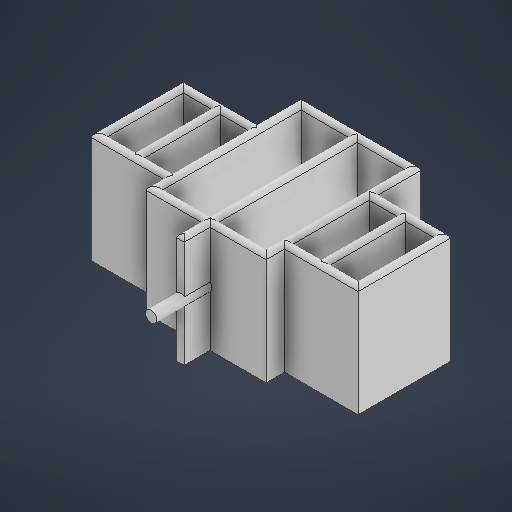
# Autodesk Inventor part: klapy
Saved by Autodesk Inventor 2026.2 (Build 302298010, 298A)
## iProperties
Created: 2026-04-21
Part Number: klapy
Material: Ogólny
Document SubType Name: Modeling
Designer: macie
Density: 1 g/cm^3
Appearance: Domyślna
Author: macie
Autodesk Inventor part; units mm, degrees
ref_plane "YZ Plane" through (0, 0, 0) normal (1, 0, 0) x (0, 1, 0)
ref_plane "XZ Plane" through (0, 0, 0) normal (0, 1, 0) x (-1, 0, 0)
ref_plane "XY Plane" through (0, 0, 0) normal (0, 0, 1) x (1, 0, 0)
sketch "Szkic1" plane through (0, 0, 0) normal (0, 1, 0) x (-1, 0, 0)
  line L0 (16.25, 0) -> (-16.25, 0)
  line L1 (-16.25, 0) -> (-16.25, 2)
  line L2 (-16.25, 2) -> (16.25, 2)
  line L3 (16.25, 2) -> (16.25, 0)
  line L4 (-1, 2) -> (1, 2)
  line L5 (1, 2) -> (1, 49)
  line L6 (1, 49) -> (-1, 49)
  line L7 (-1, 49) -> (-1, 2)
  line L8 (16.25, 2) -> (14.25, 2)
  line L9 (14.25, 2) -> (14.25, 42)
  line L10 (14.25, 42) -> (16.25, 42)
  line L11 (16.25, 42) -> (16.25, 2)
  line L12 (-16.25, 2) -> (-14.25, 2)
  line L13 (-14.25, 2) -> (-14.25, 42)
  line L14 (-14.25, 42) -> (-16.25, 42)
  line L15 (-16.25, 42) -> (-16.25, 2)
  line L16 (14.25, 42) -> (1, 42)
  line L17 (1, 42) -> (1, 40)
  line L18 (1, 40) -> (14.25, 40)
  line L19 (14.25, 40) -> (14.25, 42)
  line L20 (-14.25, 42) -> (-1, 42)
  line L21 (-1, 42) -> (-1, 40)
  line L22 (-1, 40) -> (-14.25, 40)
  line L23 (-14.25, 40) -> (-14.25, 42)
  line L24 (16.25, 37) -> (36.25, 37)
  line L25 (36.25, 37) -> (36.25, 12)
  line L26 (36.25, 12) -> (16.25, 12)
  line L27 (16.25, 12) -> (16.25, 37)
  line L28 (-16.25, 37) -> (-36.25, 37)
  line L29 (-36.25, 37) -> (-36.25, 12)
  line L30 (-36.25, 12) -> (-16.25, 12)
  line L31 (-16.25, 12) -> (-16.25, 37)
  circle A0 centre (0, -31.074) radius 80.074
  line L32 (36.25, 37) -> (34.25, 37)
  line L33 (34.25, 37) -> (34.25, 12)
  line L34 (34.25, 12) -> (36.25, 12)
  line L35 (36.25, 12) -> (36.25, 37)
  line L36 (34.25, 37) -> (16.25, 37)
  line L37 (16.25, 37) -> (16.25, 35)
  line L38 (16.25, 35) -> (34.25, 35)
  line L39 (34.25, 35) -> (34.25, 37)
  line L40 (34.25, 12) -> (16.25, 12)
  line L41 (16.25, 12) -> (16.25, 14)
  line L42 (16.25, 14) -> (34.25, 14)
  line L43 (34.25, 14) -> (34.25, 12)
  line L44 (-16.25, 37) -> (-36.25, 37)
  line L45 (-36.25, 37) -> (-36.25, 35)
  line L46 (-36.25, 35) -> (-16.25, 35)
  line L47 (-16.25, 35) -> (-16.25, 37)
  line L48 (-16.25, 12) -> (-36.25, 12)
  line L49 (-36.25, 12) -> (-36.25, 14)
  line L50 (-36.25, 14) -> (-16.25, 14)
  line L51 (-16.25, 14) -> (-16.25, 12)
  line L52 (-36.25, 35) -> (-34.25, 35)
  line L53 (-34.25, 35) -> (-34.25, 14)
  line L54 (-34.25, 14) -> (-36.25, 14)
  line L55 (-36.25, 14) -> (-36.25, 35)
  line L56 (26.25, 35) -> (24.25, 35)
  line L57 (24.25, 35) -> (24.25, 14)
  line L58 (24.25, 14) -> (26.25, 14)
  line L59 (26.25, 14) -> (26.25, 35)
  line L60 (-24.25, 35) -> (-26.25, 35)
  line L61 (-26.25, 35) -> (-26.25, 14)
  line L62 (-26.25, 14) -> (-24.25, 14)
  line L63 (-24.25, 14) -> (-24.25, 35)
  point P0 (0, 0)
  point P1 (0, 0)
  point P2 (0, 2)
  point P3 (7.625, 40)
  point P4 (7.625, 42)
  point P5 (0, 49)
  point P6 (26.25, 37)
  point P7 (26.25, 14)
  point P8 (1, 42)
  point P9 (1, 48.9938)
  point P10 (-1, 48.9938)
  point P11 (-1, 42)
  point P12 (-16.25, 12)
  point P13 (16.25, 12)
  point P14 (-16.25, 14)
  point P15 (16.25, 14)
  dimension "d0" = 32.5
  dimension "d1" = 2
  dimension "d2" = 2
  dimension "d3" = 49
  dimension "d4" = 40
  dimension "d5" = 2
  dimension "d6" = 2
  dimension "d7" = 2
  dimension "d8" = 20
  dimension "d9" = 20
  dimension "d10" = 25
  dimension "d11" = 25
  dimension "d12" = 160.148
  dimension "d13" = 80.074
  dimension "d14" = 5
  dimension "d15" = 5
  dimension "d16" = 2
  dimension "d17" = 2
  dimension "d18" = 2
  dimension "d19" = 2
  dimension "d20" = 2
  dimension "d21" = 2
  dimension "d22" = 2
  dimension "d23" = 8
  dimension "d24" = 8
  constraints: 128 end point, 32 parallel, 17 point on line, 16 horizontal, 16 perpendicular, 8 midpoint, 1 centre point, 1 coincident
  measures "d0" distance between parallel lines of L1 L3
  measures "d1" distance between parallel lines of L0 L2
  measures "d2" distance between parallel lines of L7 L5
  measures "d3" distance between parallel lines of L6 L0
  measures "d4" distance between parallel lines of L8 L10
  measures "d5" distance between parallel lines of L15 L13
  measures "d6" distance between parallel lines of L11 L9
  measures "d7" distance of point (7.625, 40) point (7.625, 42)
  measures "d8" distance between parallel lines of L11 L25
  measures "d9" distance between parallel lines of L29 L31
  measures "d10" distance between parallel lines of L24 L26
  measures "d11" distance between parallel lines of L30 L28
  measures "d12" diameter of A0
  measures "d13" distance of point (0, 49) A0.centre
  measures "d14" distance between parallel lines of L16 L24
  measures "d15" distance between parallel lines of L20 L28
  measures "d16" distance between parallel lines of L33 L25
  measures "d17" distance between parallel lines of L26 L42
  measures "d18" distance from line of point (26.25, 37) L38
  measures "d19" distance between parallel lines of L46 L28
  measures "d20" distance between parallel lines of L29 L53
  measures "d21" distance between parallel lines of L57 L59
  measures "d22" distance between parallel lines of L61 L63
  measures "d23" distance between parallel lines of L27 L57
  measures "d24" distance between parallel lines of L15 L63
extrude "Wyciągnięcie proste1" add sketch "Szkic1" along normal blind 30 contours L0 L1 L2 L3 | L2 L9 L10 L11 | L15 L14 L13 L2 | L11 L42 L33 L26 | L30 L29 L50 L15 | L2 L7 A0 L5 | L18 L5 L16 L9 | L33 L24 L25 L26 | L13 L20 L7 L22 | L11 L24 L33 L38 | L57 L38 L59 L42 | L46 L29 L28 L15 | L50 L61 L46 L63 | L29 L46 L53 L50
sketch "Szkic2" plane through (1, 0, 42) normal (0, 0, 1) x (1, 0, 0)
  circle A0 centre (-1, 15) radius 1.5
  line L0 (0, 30) -> (15.25, 30) projected
  line L1 (0, 0) -> (0, 30) projected
  point P0 (-1, 0)
  dimension "d27" = 3
  dimension "d30" = 15
  dimension "d31" = 1
  constraints: 1 centre point
  measures "d27" diameter of A0
  measures "d30" distance from line of L0 A0.centre
  measures "d31" distance from line of L1 A0.centre
extrude "Wyciągnięcie proste2" add sketch "Szkic2" along normal blind 15
fillet "Zaokrąglenie1" radius 1 40 edges at (36.25, 30, 24.5) (34.25, 30, 24.5) (26.25, 30, 37) (30.25, 30, 35) (26.25, 30, 24.5) (20.25, 30, 35) (24.25, 30, 24.5) (30.25, 30, 14) (26.25, 30, 12) (20.25, 30, 14) (1, 30, 45.4969) (0, 30, 49) (-1, 30, 45.4969) (8.625, 30, 42) (16.25, 30, 39.5) (16.25, 30, 24.5) (14.25, 30, 21) (16.25, 30, 6) (7.625, 30, 2) (0, 30, 0) (1, 30, 21) (-1, 30, 21) (7.625, 30, 40) (-7.625, 30, 40) (-8.625, 30, 42) (-16.25, 30, 39.5) (-14.25, 30, 21) (-16.25, 30, 24.5) (-26.25, 30, 37) (-20.25, 30, 35) (-24.25, 30, 24.5) (-26.25, 30, 24.5) (-30.25, 30, 35) (-34.25, 30, 24.5) (-36.25, 30, 24.5) (-30.25, 30, 14) (-26.25, 30, 12) (-20.25, 30, 14) (-16.25, 30, 6) (-7.625, 30, 2)
equation "\"d5\" = d2"
equation "\"d6\" = d2"
equation "\"d7\" = d1"
equation "\"d9\" = d8"
equation "\"d11\" = d10"
equation "\"d13\" = 0.5 * d12"
equation "\"d15\" = d14"
equation "\"d16\" = d6"
equation "\"d18\" = d17"
equation "\"d19\" = d18"
equation "\"d22\" = d21"
